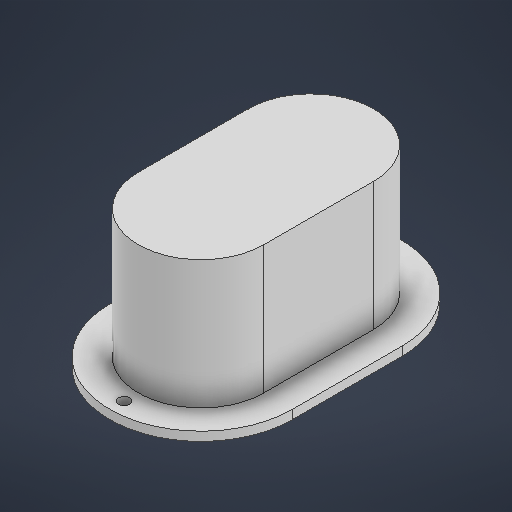
# Autodesk Inventor part: FabLabPlugwithbottom
Saved by Autodesk Inventor 2026.2 (Build 302298000, 298)
## iProperties
Created: 2026-02-11
Part Number: FabLabPlugwithbottom
Material: Generic
Document SubType Name: Modeling
Designer: 18705
Density: 1 g/cm^3
Appearance: Default
Author: 18705
Autodesk Inventor part; units mm, degrees
ref_plane "YZ Plane" through (0, 0, 0) normal (1, 0, 0) x (0, 1, 0)
ref_plane "XZ Plane" through (0, 0, 0) normal (0, 1, 0) x (-1, 0, 0)
ref_plane "XY Plane" through (0, 0, 0) normal (0, 0, 1) x (1, 0, 0)
sketch "Sketch1" plane through (0, 0, 0) normal (0, 1, 0) x (-1, 0, 0)
  line L0 (0, 12.3635) -> (0, -70.1365) construction
  line L1 (-22, -9.6365) -> (-22, -48.1365)
  line L2 (22, -48.1365) -> (22, -9.6365)
  arc A0 (22, -9.6365) -> (-22, -9.6365) centre (0, -9.6365) ccw
  arc A1 (-22, -48.1365) -> (22, -48.1365) centre (0, -48.1365) ccw
  point P0 (0, 0)
  point P1 (0, -28.8865)
  dimension "d0" = 82.5
  dimension "d1" = 44
  constraints: 8 end point, 6 point on circle, 4 tangent, 2 centre point, 2 point on line, 1 midpoint, 1 parallel, 1 vertical
  measures "d0" distance of L0.start L0.end
  measures "d1" diameter of A1
extrude "Extrusion1" add sketch "Sketch1" along normal blind 45
sketch "Sketch2" plane through (0, 0, 0) normal (0, -1, 0) x (1, 0, 0)
  arc A0 (22, -9.6365) -> (-22, -9.6365) centre (0, -9.6365) ccw projected
  line L0 (0, 12.3635) -> (0, -70.1365)
  arc A1 (-22, -48.1365) -> (22, -48.1365) centre (0, -48.1365) ccw projected
  line L1 (0, -28.8865) -> (22, -28.8865) construction
  line L2 (0, 22.3635) -> (0, -80.1365) construction
  line L3 (-32, -9.6365) -> (-32, -48.1365)
  line L4 (32, -48.1365) -> (32, -9.6365)
  arc A2 (32, -9.6365) -> (-32, -9.6365) centre (0, -9.6365) ccw
  arc A3 (-32, -48.1365) -> (32, -48.1365) centre (0, -48.1365) ccw
  line L5 (22, -9.6365) -> (22, -48.1365) projected
  line L6 (-22, -48.1365) -> (-22, -9.6365) projected
  point P0 (0, 0)
  point P1 (8.1717, -6.5277)
  point P2 (0, -80.1365)
  point P3 (0, 22.3635)
  point P4 (0, -70.1365)
  dimension "d8" = 10
  dimension "d9" = 10
  dimension "d10" = 10
  constraints: 12 end point, 11 point on circle, 4 tangent, 2 centre point, 2 midpoint, 2 point on line, 2 vertical, 1 coincident, 1 horizontal, 1 parallel
  measures "d8" distance between parallel lines of L4 L5
  measures "d9" distance between parallel lines of L3 L6
  measures "d10" distance of L2.end point (0, -70.137)
extrude "Extrusion2" add sketch "Sketch2" along normal blind 3.11 contours L5 A1 L0 A0 | L0 A1 L6 A0 | A2 L4 A3 L3
sketch "Sketch3" plane through (0, 0, 0) normal (0, 1, 0) x (1, 0, 0)
  circle A0 centre (0, -17.3635) radius 2
  arc A1 (-22, 9.6365) -> (22, 9.6365) centre (0, 9.6365) ccw projected
  line L0 (-32, 9.6365) -> (-32, 48.1365) projected
  line L1 (-32, 28.8865) -> (32, 28.8865) construction
  line L2 (32, 48.1365) -> (32, 9.6365) projected
  circle A2 centre (0, 75.1365) radius 2
  point P0 (0, 0)
  point P1 (0, -12.3635)
  dimension "d13" = 4
  dimension "d14" = 5
  constraints: 2 centre point, 2 end point, 2 midpoint, 1 point on circle, 1 symmetric about line, 1 other
  measures "d13" diameter of A0
  measures "d14" distance of point (0, -12.363) A0.centre
extrude "Extrusion3" cut sketch "Sketch3" against normal blind 7.7
body "Solid1"
